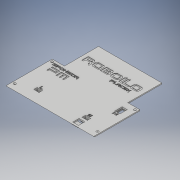
# Autodesk Inventor part: dach
Saved by Autodesk Inventor 2019 (Build 230136000, 136)
## iProperties
Created: 2019-09-08
Part Number: dach
Material: Generic
Document SubType Name: Modeling
Designer: Michal
Density: 1 g/cm^3
Appearance: Default
Author: Michal
Autodesk Inventor part; units mm, degrees
ref_plane "YZ Plane" through (0, 0, 0) normal (1, 0, 0) x (0, 1, 0)
ref_plane "XZ Plane" through (0, 0, 0) normal (0, 1, 0) x (-1, 0, 0)
ref_plane "XY Plane" through (0, 0, 0) normal (0, 0, 1) x (1, 0, 0)
sketch "Sketch1" plane through (0, 0, 0) normal (0, 1, 0) x (-1, 0, 0)
  line L0 (0, 0) -> (180, 0)
  line L1 (180, 0) -> (180, -95)
  line L2 (0, 0) -> (0, -95)
  line L3 (180, -95) -> (155, -95)
  line L4 (0, -95) -> (25, -95)
  line L5 (25, -95) -> (25, -165)
  line L6 (155, -95) -> (155, -165)
  line L7 (155, -165) -> (25, -165)
  dimension "d0" = 180
  dimension "d1" = 95
  dimension "d4" = 95
  dimension "d35" = 25
  dimension "d36" = 25
  constraints: 16 end point, 4 horizontal, 2 perpendicular, 2 vertical
  measures "d0" distance of L0.start L0.end
  measures "d1" distance of L0.end L1.end
  measures "d4" distance of L0.start L2.end
  measures "d35" distance of L1.end L3.end
  measures "d36" distance of L2.end L4.end
extrude "Extrusion1" add sketch "Sketch1" along normal blind 2
sketch "Sketch3" plane through (-155, 0, -165) normal (-1, 0, 0) x (0, 0, 1)
  line L0 (70, 2) -> (0, 2) projected
  line L1 (0, 2) -> (28, 2)
  line L2 (28, 2) -> (28, -13)
  circle A0 centre (28, -13) radius 12.5
  point P0 (165, 0)
  dimension "d46" = 28
  dimension "d47" = 15
  dimension "d48" = 25
  constraints: 4 end point, 1 centre point, 1 coincident, 1 perpendicular, 1 point on line
  measures "d46" distance of L0.end L1.end
  measures "d47" distance of L1.end L2.end
  measures "d48" diameter of A0
extrude "Extrusion3" cut sketch "Sketch3" against normal blind 130
chamfer "Chamfer1" distance 2 angle 45 1 edges at (-90, 0, 0)
sketch "Sketch7" plane through (0, 2, 0) normal (0, 1, 0) x (1, 0, 0)
  line L0 (-155, 95) -> (-180, 95) projected
  line L1 (-180, 95) -> (-175, 95)
  line L2 (-175, 95) -> (-175, 90)
  line L3 (-175, 90) -> (-180, 90)
  line L4 (-180, 90) -> (-180, 95)
  line L5 (0, 95) -> (-25, 95) projected
  line L6 (0, 95) -> (-5, 95)
  line L7 (-5, 95) -> (-5, 90)
  line L8 (-5, 90) -> (0, 90)
  line L9 (0, 90) -> (0, 95)
  line L10 (-5, 90) -> (-5, 13)
  line L11 (-175, 90) -> (-175, 13)
  point P0 (0, 0)
  dimension "d80" = 5
  dimension "d81" = 5
  dimension "d82" = 5
  dimension "d83" = 77
  constraints: 20 end point, 4 parallel, 2 horizontal, 2 perpendicular, 2 vertical, 1 point on line
  measures "d80" distance of L2.end L3.end
  measures "d81" distance of L1.end L2.end
  measures "d82" distance of L8.end L7.end
  measures "d83" distance of L7.end L10.end
hole "Hole1" at (-175, 2, -90) at (-5, 2, -90) at (-5, 2, -13) at (-175, 2, -13) direction (0, -1, 0) diameter 2.4638 depth 8.7884 countersink diameter 5 countersink angle 75
sketch "Sketch8" plane through (0, 2, 0) normal (0, 1, 0) x (1, 0, 0)
  line L0 (0, 0) -> (0, 95) projected
  line L1 (0, 95) -> (-13, 95)
  line L2 (-13, 95) -> (-13, 82)
  line L3 (-13, 82) -> (0, 82)
  line L4 (0, 82) -> (0, 95)
  line L5 (-13, 82) -> (-23.5, 82)
  line L6 (-23.5, 82) -> (-23.5, 67)
  line L7 (-23.5, 67) -> (-13, 67)
  line L8 (-13, 67) -> (-13, 82)
  line L9 (-180, 95) -> (-180, 0) projected
  line L10 (-180, 0) -> (0, 0) projected
  line L11 (0, 0) -> (-35, 0)
  line L12 (-35, 0) -> (-35, 4)
  line L13 (-35, 4) -> (0, 4)
  line L14 (0, 4) -> (0, 0)
  line L15 (-35, 4) -> (-47, 4)
  line L16 (-47, 4) -> (-47, 17)
  line L17 (-47, 17) -> (-35, 17)
  line L18 (-35, 17) -> (-35, 4)
  line L19 (-35, 17) -> (-35, 22)
  line L20 (-35, 22) -> (-46, 22)
  line L21 (-46, 22) -> (-46, 29)
  line L22 (-46, 29) -> (-35, 29)
  line L23 (-35, 29) -> (-35, 22)
  line L24 (-180, 0) -> (-145, 0)
  line L25 (-145, 0) -> (-145, 22)
  line L26 (-145, 22) -> (-180, 22)
  line L27 (-180, 22) -> (-180, 0)
  line L28 (-145, 22) -> (-134, 22)
  line L29 (-134, 22) -> (-134, 29)
  line L30 (-134, 29) -> (-145, 29)
  line L31 (-145, 29) -> (-145, 22)
  dimension "d91" = 13
  dimension "d92" = 13
  dimension "d93" = 10.5
  dimension "d94" = 15
  dimension "d128" = 35
  dimension "d129" = 4
  dimension "d130" = 12
  dimension "d131" = 13
  dimension "d141" = 5
  dimension "d142" = 11
  dimension "d143" = 7
  dimension "d158" = 35
  dimension "d159" = 22
  dimension "d160" = 11
  dimension "d161" = 7
  constraints: 58 end point, 14 parallel, 7 horizontal, 7 perpendicular, 1 vertical
  measures "d91" distance of L3.end L2.end
  measures "d92" distance of L2.end L1.end
  measures "d93" distance of L7.end L6.end
  measures "d94" distance of L6.end L5.end
  measures "d128" distance of L12.end L13.end
  measures "d129" distance of L11.end L12.end
  measures "d130" distance of L16.end L17.end
  measures "d131" distance of L15.end L16.end
  measures "d141" distance of L17.end L19.end
  measures "d142" distance of L21.end L22.end
  measures "d143" distance of L20.end L21.end
  measures "d158" distance of L26.end L25.end
  measures "d159" distance of L25.end L24.end
  measures "d160" distance of L30.end L29.end
  measures "d161" distance of L29.end L28.end
extrude "Extrusion7" cut sketch "Sketch8" against normal blind 2 contours L15 L16 L17 L18 | L8 L7 L6 L5 | L31 L30 L29 L28 | L20 L21 L22 L23
sketch "Sketch9" plane through (0, 0, 0) normal (0, -1, 0) x (1, 0, 0)
  line L0 (-13, -67) -> (-23.5, -67) projected
  line L1 (-23.5, -67) -> (-23.5, -82) projected
  line L2 (-13, -67) -> (-23.5, -67)
  line L3 (-23.5, -67) -> (-23.5, -82)
  line L4 (-23.5, -82) -> (-13, -82)
  line L5 (-13, -82) -> (-13, -67)
  line L6 (-23.5, -82) -> (-13, -82) projected
  line L7 (-11, -65) -> (-25.5, -65)
  line L8 (-25.5, -65) -> (-25.5, -84)
  line L9 (-25.5, -84) -> (-11, -84)
  line L10 (-11, -84) -> (-11, -65)
  point P0 (0, 0)
  constraints: 16 end point, 4 parallel, 2 horizontal, 2 perpendicular
extrude "Extrusion8" add sketch "Sketch9" along normal blind 3
sketch "Sketch10" plane through (-13, 2, -82) normal (-1, 0, 0) x (0, 0, 1)
  line L0 (0, 0) -> (15, 0) projected
  line L1 (0, 0) -> (0, -3)
  line L2 (0, 0) -> (0, -5) projected
  line L3 (15, 0) -> (15, -5) projected
  line L4 (0, -3) -> (15, -3)
  line L5 (15, -3) -> (15, -5)
  line L6 (15, -5) -> (0, -5)
  line L7 (0, -5) -> (0, -3)
  point P0 (82, -2)
  dimension "d103" = 3
  constraints: 10 end point, 2 parallel, 1 horizontal, 1 perpendicular, 1 point on line
  measures "d103" distance of L0.start L1.end
extrude "Extrusion9" add sketch "Sketch10" along normal blind 1 contours L4 L3 L6 L2
sketch "Sketch11" plane through (-23.5, 2, -67) normal (1, 0, 0) x (0, 0, -1)
  line L0 (15, 0) -> (15, -3) projected
  line L1 (15, 0) -> (15, -3)
  line L2 (0, -3) -> (15, -3) projected
  line L3 (15, -5) -> (0, -5) projected
  line L4 (15, -3) -> (0, -3)
  line L5 (0, -3) -> (0, -5)
  line L6 (0, -5) -> (15, -5)
  line L7 (15, -5) -> (15, -3)
  point P0 (-67, -2)
  constraints: 10 end point, 2 parallel, 1 horizontal, 1 perpendicular, 1 vertical
extrude "Extrusion10" add sketch "Sketch11" along normal blind 1
sketch "Sketch12" plane through (-23.5, 2, -82) normal (0, 0, 1) x (1, 0, 0)
  line L0 (9.5, -3) -> (9.5, -5) projected
  line L1 (1, -3) -> (0, -3) projected
  line L2 (9.5, -5) -> (1, -5)
  line L3 (1, -5) -> (1, -3)
  line L4 (1, -3) -> (9.5, -3)
  line L5 (9.5, -3) -> (9.5, -5)
  point P0 (23.5, -2)
  constraints: 8 end point, 2 parallel, 1 horizontal, 1 perpendicular
extrude "Extrusion11" add sketch "Sketch12" along normal blind 1.3
sketch "Sketch13" plane through (-13, 2, -67) normal (0, 0, -1) x (-1, 0, 0)
  line L0 (0, -3) -> (1, -3) projected
  line L1 (-2, -5) -> (12.5, -5) projected
  line L2 (0, -3) -> (10.5024, -3)
  line L3 (10.5024, -3) -> (10.5024, -5)
  line L4 (10.5024, -5) -> (0, -5)
  line L5 (0, -5) -> (0, -3)
  point P0 (-13, -2)
  constraints: 8 end point, 2 parallel, 1 horizontal, 1 perpendicular, 1 point on line
extrude "Extrusion12" add sketch "Sketch13" along normal blind 1.3
sketch "Sketch14" plane through (0, -3, 0) normal (0, -1, 0) x (1, 0, 0)
  line L0 (-22.5, -68.3) -> (-22.5, -67)
  line L1 (-13, -67) -> (-23.5, -67) projected
  line L2 (-22.5, -67) -> (-14, -67)
  line L3 (-22.5, -68.3) -> (-14, -68.3) projected
  line L4 (-14, -67) -> (-14, -68.3)
  line L5 (-14, -68.3) -> (-22.5, -68.3)
  line L6 (-22.5, -80.7) -> (-22.5, -68.3) projected
  line L7 (-22.5, -80.7) -> (-22.5, -82)
  line L8 (-23.5, -82) -> (-13, -82) projected
  line L9 (-14, -80.7) -> (-22.5, -80.7) projected
  line L10 (-22.5, -80.7) -> (-14, -80.7)
  line L11 (-14, -80.7) -> (-14, -82)
  line L12 (-14, -82) -> (-22.5, -82)
  point P0 (0, 0)
  constraints: 16 end point, 3 perpendicular, 2 collinear, 2 point on line, 2 vertical, 1 horizontal
extrude "Extrusion13" cut sketch "Sketch14" against normal blind 1
sketch "Sketch17" plane through (0, 0, 0) normal (0, -1, 0) x (1, 0, 0)
  line L0 (-47, -4) -> (-35, -4) projected
  line L1 (-35, -17) -> (-47, -17) projected
  line L2 (-35, -4) -> (-47, -4)
  line L3 (-47, -4) -> (-47, -17)
  line L4 (-47, -17) -> (-35, -17)
  line L5 (-35, -17) -> (-35, -4)
  line L6 (-34, -4) -> (-34, -3)
  line L7 (-34, -3) -> (-35, -3)
  line L8 (-48, -17) -> (-48, -18)
  line L9 (-48, -18) -> (-47, -18)
  line L10 (-48, -18) -> (-34, -18)
  line L11 (-34, -18) -> (-34, -3)
  line L12 (-34, -3) -> (-48, -3)
  line L13 (-48, -3) -> (-48, -18)
  point P0 (0, 0)
  dimension "d132" = 1
  dimension "d133" = 1
  dimension "d134" = 1
  dimension "d135" = 1
  constraints: 24 end point, 4 parallel, 2 horizontal, 2 perpendicular
  measures "d132" distance of L7.end L6.end
  measures "d133" distance of L6.end L6.start
  measures "d134" distance of L9.end L8.end
  measures "d135" distance of L8.end L8.start
extrude "Extrusion16" add sketch "Sketch17" along normal blind 0.5
sketch "Sketch18" plane through (0, -0.5, 0) normal (0, -1, 0) x (1, 0, 0)
  line L0 (-34, -3) -> (-48, -3) projected
  line L1 (-34, -18) -> (-34, -3) projected
  line L2 (-48, -3) -> (-34, -3)
  line L3 (-34, -3) -> (-34, -13)
  line L4 (-34, -13) -> (-48, -13)
  line L5 (-48, -13) -> (-48, -3)
  point P0 (0, 0)
  dimension "d138" = 10
  constraints: 8 end point, 2 parallel, 1 horizontal, 1 perpendicular, 1 point on line
  measures "d138" distance of L2.end L3.end
extrude "Extrusion17" add sketch "Sketch18" along normal blind 1
sketch "Sketch19" plane through (0, 0, 0) normal (0, -1, 0) x (1, 0, 0)
  line L0 (-46, -22) -> (-35, -22) projected
  line L1 (-35, -22) -> (-46, -22)
  line L2 (-46, -22) -> (-46, -29)
  line L3 (-46, -29) -> (-35, -29)
  line L4 (-35, -29) -> (-35, -22)
  line L5 (-47, -30) -> (-34, -30)
  line L6 (-34, -30) -> (-34, -21)
  line L7 (-34, -21) -> (-47, -21)
  line L8 (-47, -21) -> (-47, -30)
  line L9 (-134, -22) -> (-145, -22)
  line L10 (-145, -22) -> (-145, -29)
  line L11 (-145, -29) -> (-134, -29)
  line L12 (-134, -29) -> (-134, -22)
  line L13 (-146, -30) -> (-133, -30)
  line L14 (-133, -30) -> (-133, -21)
  line L15 (-133, -21) -> (-146, -21)
  line L16 (-146, -21) -> (-146, -30)
  point P0 (0, 0)
  constraints: 32 end point, 8 parallel, 4 horizontal, 4 perpendicular
extrude "Extrusion18" add sketch "Sketch19" along normal blind 4
sketch "Sketch20" plane through (0, -4, 0) normal (0, -1, 0) x (1, 0, 0)
  line L0 (-34, -30) -> (-47, -30) projected
  line L1 (-47, -21) -> (-34, -21) projected
  line L2 (-34, -30) -> (-47, -30)
  line L3 (-47, -30) -> (-47, -21)
  line L4 (-47, -21) -> (-34, -21)
  line L5 (-34, -21) -> (-34, -30)
  line L6 (-46, -22) -> (-46, -29) projected
  line L7 (-46, -29) -> (-35, -29) projected
  line L8 (-46, -22) -> (-42, -22)
  line L9 (-42, -22) -> (-42, -29)
  line L10 (-42, -29) -> (-46, -29)
  line L11 (-46, -29) -> (-46, -22)
  line L12 (-35, -22) -> (-46, -22) projected
  line L13 (-35, -29) -> (-39, -29)
  line L14 (-39, -29) -> (-39, -22)
  line L15 (-39, -22) -> (-35, -22)
  line L16 (-35, -22) -> (-35, -29)
  line L17 (-133, -30) -> (-146, -30) projected
  line L18 (-133, -30) -> (-146, -30)
  line L19 (-146, -30) -> (-146, -21)
  line L20 (-146, -21) -> (-133, -21)
  line L21 (-133, -21) -> (-133, -30)
  line L22 (-145, -22) -> (-141, -22)
  line L23 (-141, -22) -> (-141, -29)
  line L24 (-141, -29) -> (-145, -29)
  line L25 (-145, -29) -> (-145, -22)
  line L26 (-134, -29) -> (-138, -29)
  line L27 (-138, -29) -> (-138, -22)
  line L28 (-138, -22) -> (-134, -22)
  line L29 (-134, -22) -> (-134, -29)
  point P0 (0, 0)
  dimension "d150" = 4
  dimension "d151" = 4
  dimension "d162" = 4
  dimension "d163" = 4
  constraints: 48 end point, 12 parallel, 6 horizontal, 6 perpendicular, 2 point on line
  measures "d150" distance of L9.end L10.end
  measures "d151" distance of L14.end L15.end
  measures "d162" distance of L23.end L25.start
  measures "d163" distance of L28.start L29.start
extrude "Extrusion19" add sketch "Sketch20" along normal blind 1.5 contours L0 L3 L1 L5 | L12 L14 L7 L9 | L17 L19 L20 L21
sketch "Sketch5" plane through (0, 2, 0) normal (0, 1, 0) x (1, 0, 0)
  line L0 (-154.7367, 165.2131) -> (-24.9468, 165.2131) construction
  line L1 (-24.9468, 165.2131) -> (-24.9468, 95.1481) construction
  line L2 (-24.9468, 95.1481) -> (-154.7367, 95.1481) construction
  line L3 (-154.7367, 95.1481) -> (-154.7367, 165.2131) construction
  line L4 (-82.3644, 120.7847) -> (-41.6119, 120.7847) construction
  line L5 (-41.6119, 120.7847) -> (-41.6119, 113.7771) construction
  line L6 (-41.6119, 113.7771) -> (-82.3644, 113.7771) construction
  line L7 (-82.3644, 113.7771) -> (-82.3644, 120.7847) construction
  line L8 (-44.6378, 36.0437) -> (-36.7668, 36.0437) construction
  line L9 (-36.7668, 36.0437) -> (-36.7668, 30.8473) construction
  line L10 (-36.7668, 30.8473) -> (-44.6378, 30.8473) construction
  line L11 (-44.6378, 30.8473) -> (-44.6378, 36.0437) construction
  line L12 (-22.1506, 65.5798) -> (-13.2194, 65.5798) construction
  line L13 (-13.2194, 65.5798) -> (-13.2194, 59.4838) construction
  line L14 (-13.2194, 59.4838) -> (-22.1506, 59.4838) construction
  line L15 (-22.1506, 59.4838) -> (-22.1506, 65.5798) construction
  line L16 (-142.4189, 36.7707) -> (-136.2064, 36.7707) construction
  line L17 (-136.2064, 36.7707) -> (-136.2064, 30.6546) construction
  line L18 (-136.2064, 30.6546) -> (-142.4189, 30.6546) construction
  line L19 (-142.4189, 30.6546) -> (-142.4189, 36.7707) construction
  line L20 (-180, 2) -> (-180, 95) projected
  line L21 (-166.0933, 81.4189) -> (-150.8913, 81.4189)
  line L22 (-150.8913, 81.4189) -> (-150.8913, 72.9559)
  line L23 (-166.0933, 81.4189) -> (-166.0933, 78.7799)
  line L24 (-166.0933, 78.7799) -> (-153.5243, 78.7799)
  line L25 (-153.5243, 78.7799) -> (-153.5243, 75.5879)
  line L26 (-153.5243, 75.5879) -> (-166.0933, 75.5879)
  line L27 (-166.0933, 75.5879) -> (-166.0933, 69.8939)
  line L28 (-166.0933, 69.8939) -> (-163.4573, 69.8939)
  line L29 (-163.4573, 69.8939) -> (-163.4573, 72.9559)
  line L30 (-163.4573, 72.9559) -> (-150.8913, 72.9559)
  line L31 (-150.8913, 81.4189) -> (-147.5843, 81.4189)
  line L32 (-147.5843, 81.4189) -> (-147.5843, 69.8939)
  line L33 (-147.5843, 69.8939) -> (-144.9503, 69.8939)
  line L34 (-144.9503, 69.8939) -> (-144.9503, 78.7799)
  line L35 (-144.9503, 78.7799) -> (-133.8883, 78.7799)
  line L36 (-133.8883, 78.7799) -> (-133.8883, 69.8939)
  line L37 (-133.8883, 69.8939) -> (-131.2543, 69.8939)
  line L38 (-131.2543, 69.8939) -> (-131.2543, 81.4189)
  line L39 (-131.2543, 81.4189) -> (-147.5843, 81.4189)
  line L40 (-144.9503, 78.7799) -> (-140.7343, 78.7799)
  line L41 (-133.8883, 78.7799) -> (-138.1043, 78.7799)
  line L42 (-138.1043, 78.7799) -> (-138.1043, 77.2269)
  line L43 (-138.1043, 77.2269) -> (-140.7343, 77.2269)
  line L44 (-140.7343, 77.2269) -> (-140.7343, 69.8939)
  line L45 (-140.7343, 69.8939) -> (-138.1043, 69.8939)
  line L46 (-138.1043, 69.8939) -> (-138.1043, 77.2269)
  line L47 (-170.8643, 90.9845) -> (-118.0724, 90.9845) construction
  line L48 (-118.0724, 90.9845) -> (-118.0724, 83.2717) construction
  line L49 (-118.0724, 83.2717) -> (-170.8643, 83.2717) construction
  line L50 (-170.8643, 83.2717) -> (-170.8643, 90.9845) construction
  line L51 (-75.7423, 118.2788) -> (-77.1197, 116.4155)
  line L52 (-77.1197, 116.4155) -> (-80.7902, 116.4155)
  line L53 (-80.7902, 116.4155) -> (-80.7902, 113.7771)
  line L54 (-80.7902, 113.7771) -> (-82.3604, 114.6766)
  line L55 (-82.3604, 114.6766) -> (-82.3604, 119.8731)
  line L56 (-82.3604, 119.8731) -> (-76.927, 119.8731)
  line L57 (-76.927, 119.8731) -> (-75.7423, 118.2788)
  line L58 (-77.3607, 118.1704) -> (-77.7743, 118.7165)
  line L59 (-77.7743, 118.7165) -> (-80.7902, 118.7165)
  line L60 (-80.7902, 118.7165) -> (-80.7902, 117.5961)
  line L61 (-80.7902, 117.5961) -> (-77.7743, 117.5961)
  line L62 (-77.7743, 117.5961) -> (-77.3607, 118.1704)
  line L63 (-69.1925, 115.8332) -> (-70.3571, 114.6686)
  line L64 (-70.3571, 114.6686) -> (-75.2283, 114.6686)
  line L65 (-75.2283, 114.6686) -> (-75.2283, 119.8771)
  line L66 (-75.2283, 119.8771) -> (-73.6581, 120.7847)
  line L67 (-73.6581, 120.7847) -> (-73.6581, 115.8332)
  line L68 (-73.6581, 115.8332) -> (-69.1925, 115.8332)
  line L69 (-62.707, 113.7771) -> (-64.2852, 114.6686)
  line L70 (-64.2852, 114.6686) -> (-64.2852, 116.1665)
  line L71 (-64.2852, 116.1665) -> (-67.4456, 116.1665)
  line L72 (-67.4456, 116.1665) -> (-67.4456, 114.6686)
  line L73 (-67.4456, 114.6686) -> (-69.0158, 114.6766)
  line L74 (-69.0158, 114.6766) -> (-69.0158, 118.7085)
  line L75 (-69.0158, 118.7085) -> (-67.8352, 119.8731)
  line L76 (-67.8352, 119.8731) -> (-63.8876, 119.8731)
  line L77 (-63.8876, 119.8731) -> (-62.707, 118.7085)
  line L78 (-62.707, 118.7085) -> (-62.707, 113.7771)
  line L79 (-64.2852, 117.315) -> (-64.2852, 118.7085)
  line L80 (-64.2852, 118.7085) -> (-67.4456, 118.7085)
  line L81 (-67.4456, 118.7085) -> (-67.4456, 117.315)
  line L82 (-67.4456, 117.315) -> (-64.2852, 117.315)
  line L83 (-55.5789, 119.8731) -> (-56.7355, 118.7085)
  line L84 (-56.7355, 118.7085) -> (-60.2292, 118.7085)
  line L85 (-60.2292, 118.7085) -> (-60.2292, 115.8332)
  line L86 (-60.2292, 115.8332) -> (-55.7636, 115.8332)
  line L87 (-55.7636, 115.8332) -> (-56.9282, 114.6686)
  line L88 (-56.9282, 114.6686) -> (-60.6188, 114.6686)
  line L89 (-60.6188, 114.6686) -> (-61.7994, 115.8332)
  line L90 (-61.7994, 115.8332) -> (-61.7994, 118.6844)
  line L91 (-61.7994, 118.6844) -> (-60.6188, 119.8731)
  line L92 (-60.6188, 119.8731) -> (-55.5789, 119.8731)
  line L93 (-49.005, 119.8731) -> (-50.1616, 118.7085)
  line L94 (-50.1616, 118.7085) -> (-53.6553, 118.7085)
  line L95 (-53.6553, 118.7085) -> (-53.6553, 117.8009)
  line L96 (-53.6553, 117.8009) -> (-49.764, 117.8009)
  line L97 (-49.764, 117.8009) -> (-50.8242, 116.7407)
  line L98 (-50.8242, 116.7407) -> (-53.6553, 116.7407)
  line L99 (-53.6553, 116.7407) -> (-53.6553, 115.8332)
  line L100 (-53.6553, 115.8332) -> (-49.1898, 115.8332)
  line L101 (-49.1898, 115.8332) -> (-50.3544, 114.6686)
  line L102 (-50.3544, 114.6686) -> (-55.2255, 114.6686)
  line L103 (-55.2255, 114.6686) -> (-55.2255, 119.8731)
  line L104 (-55.2255, 119.8731) -> (-49.005, 119.8731)
  line L105 (-42.3549, 119.8731) -> (-44.3347, 117.9816)
  line L106 (-44.3347, 117.9816) -> (-42.5195, 116.1665)
  line L107 (-42.5195, 116.1665) -> (-42.5195, 114.6686)
  line L108 (-42.5195, 114.6686) -> (-44.0897, 113.7771)
  line L109 (-44.0897, 113.7771) -> (-44.0897, 115.9376)
  line L110 (-44.0897, 115.9376) -> (-45.2503, 117.0981)
  line L111 (-45.2503, 117.0981) -> (-46.9208, 115.528)
  line L112 (-46.9208, 115.528) -> (-46.9208, 114.6686)
  line L113 (-46.9208, 114.6686) -> (-48.491, 114.6766)
  line L114 (-48.491, 114.6766) -> (-48.491, 119.8731)
  line L115 (-48.491, 119.8731) -> (-46.9208, 119.8731)
  line L116 (-46.9208, 119.8731) -> (-46.9208, 117.323)
  line L117 (-46.9208, 117.323) -> (-44.2102, 119.8731)
  line L118 (-44.2102, 119.8731) -> (-42.3549, 119.8731)
  line L119 (-131.1694, 121.4211) -> (-135.0949, 123.67)
  line L120 (-135.0949, 123.67) -> (-135.0949, 126.8525)
  line L121 (-135.0949, 126.8525) -> (-136.2896, 128.0171)
  line L122 (-136.2896, 128.0171) -> (-143.7891, 128.0171)
  line L123 (-143.7891, 128.0171) -> (-143.7891, 123.67)
  line L124 (-143.7891, 123.67) -> (-147.7146, 123.67)
  line L125 (-147.7146, 123.67) -> (-147.7146, 136.6611)
  line L126 (-147.7146, 136.6611) -> (-134.1311, 136.6611)
  line L127 (-134.1311, 136.6611) -> (-131.1694, 132.6754)
  line L128 (-131.1694, 132.6754) -> (-133.4183, 129.6535)
  line L129 (-133.4183, 129.6535) -> (-131.1694, 127.3946)
  line L130 (-131.1694, 127.3946) -> (-131.1694, 121.4211)
  line L131 (-135.2053, 132.4044) -> (-136.2494, 133.7697)
  line L132 (-136.2494, 133.7697) -> (-143.7891, 133.7697)
  line L133 (-143.7891, 133.7697) -> (-143.7891, 130.9687)
  line L134 (-143.7891, 130.9687) -> (-136.2595, 130.9687)
  line L135 (-136.2595, 130.9687) -> (-135.2053, 132.4044)
  line L136 (-112.1947, 126.6216) -> (-115.1464, 123.67)
  line L137 (-115.1464, 123.67) -> (-125.989, 123.67)
  line L138 (-125.989, 123.67) -> (-128.9407, 126.6216)
  line L139 (-128.9407, 126.6216) -> (-128.9407, 133.7095)
  line L140 (-128.9407, 133.7095) -> (-125.989, 136.6611)
  line L141 (-125.989, 136.6611) -> (-115.1464, 136.6611)
  line L142 (-115.1464, 136.6611) -> (-112.1947, 133.7095)
  line L143 (-112.1947, 133.7095) -> (-112.1947, 126.6216)
  line L144 (-116.1202, 126.5614) -> (-116.1202, 133.7697)
  line L145 (-116.1202, 133.7697) -> (-125.0152, 133.7697)
  line L146 (-125.0152, 133.7697) -> (-125.0152, 126.5614)
  line L147 (-125.0152, 126.5614) -> (-116.1202, 126.5614)
  line L148 (-93.3807, 127.6456) -> (-96.3323, 123.6499)
  line L149 (-96.3323, 123.6499) -> (-110.0965, 123.6499)
  line L150 (-110.0965, 123.6499) -> (-110.0965, 136.6611)
  line L151 (-110.0965, 136.6611) -> (-96.3323, 136.6611)
  line L152 (-96.3323, 136.6611) -> (-93.3807, 132.6654)
  line L153 (-93.3807, 132.6654) -> (-95.2279, 130.1555)
  line L154 (-95.2279, 130.1555) -> (-93.3807, 127.6456)
  line L155 (-97.6776, 127.6456) -> (-98.6313, 128.8303)
  line L156 (-98.6313, 128.8303) -> (-106.171, 128.8303)
  line L157 (-106.171, 128.8303) -> (-106.171, 126.5614)
  line L158 (-106.171, 126.5614) -> (-98.6313, 126.5614)
  line L159 (-98.6313, 126.5614) -> (-97.6776, 127.6456)
  line L160 (-97.6776, 132.6654) -> (-98.6313, 133.7497)
  line L161 (-98.6313, 133.7497) -> (-106.171, 133.7497)
  line L162 (-106.171, 133.7497) -> (-106.171, 131.4807)
  line L163 (-106.171, 131.4807) -> (-98.6313, 131.4807)
  line L164 (-98.6313, 131.4807) -> (-97.6776, 132.6654)
  line L165 (-74.5766, 126.6216) -> (-77.5283, 123.67)
  line L166 (-77.5283, 123.67) -> (-88.3709, 123.67)
  line L167 (-88.3709, 123.67) -> (-91.3226, 126.6216)
  line L168 (-91.3226, 126.6216) -> (-91.3226, 133.7095)
  line L169 (-91.3226, 133.7095) -> (-88.3709, 136.6611)
  line L170 (-88.3709, 136.6611) -> (-77.5283, 136.6611)
  line L171 (-77.5283, 136.6611) -> (-74.5766, 133.7095)
  line L172 (-74.5766, 133.7095) -> (-74.5766, 126.6216)
  line L173 (-78.5021, 126.5614) -> (-78.5021, 133.7697)
  line L174 (-78.5021, 133.7697) -> (-87.3971, 133.7697)
  line L175 (-87.3971, 133.7697) -> (-87.3971, 126.5614)
  line L176 (-87.3971, 126.5614) -> (-78.5021, 126.5614)
  line L177 (-68.5529, 123.6499) -> (-72.4784, 123.67)
  line L178 (-72.4784, 123.67) -> (-72.4784, 136.6712)
  line L179 (-72.4784, 136.6712) -> (-68.5529, 138.9401)
  line L180 (-68.5529, 138.9401) -> (-68.5529, 123.6499)
  line L181 (-51.2347, 126.5614) -> (-54.1462, 123.6499)
  line L182 (-54.1462, 123.6499) -> (-66.3241, 123.6499)
  line L183 (-66.3241, 123.6499) -> (-66.3241, 136.6712)
  line L184 (-66.3241, 136.6712) -> (-62.3987, 138.9401)
  line L185 (-62.3987, 138.9401) -> (-62.3987, 126.5614)
  line L186 (-62.3987, 126.5614) -> (-51.2347, 126.5614)
  line L187 (-34.0471, 126.6216) -> (-36.9987, 123.67)
  line L188 (-36.9987, 123.67) -> (-47.8414, 123.67)
  line L189 (-47.8414, 123.67) -> (-50.793, 126.6216)
  line L190 (-50.793, 126.6216) -> (-50.793, 133.7095)
  line L191 (-50.793, 133.7095) -> (-47.8414, 136.6611)
  line L192 (-47.8414, 136.6611) -> (-36.9987, 136.6611)
  line L193 (-36.9987, 136.6611) -> (-34.0471, 133.7095)
  line L194 (-34.0471, 133.7095) -> (-34.0471, 126.6216)
  line L195 (-37.9725, 126.5614) -> (-37.9725, 133.7697)
  line L196 (-37.9725, 133.7697) -> (-46.8675, 133.7697)
  line L197 (-46.8675, 133.7697) -> (-46.8675, 126.5614)
  line L198 (-46.8675, 126.5614) -> (-37.9725, 126.5614)
  line L199 (-14.0989, 60.3834) -> (-15.6691, 60.3834)
  line L200 (-15.6691, 60.3834) -> (-15.6691, 63.7085)
  line L201 (-15.6691, 63.7085) -> (-17.6207, 61.0299)
  line L202 (-17.6207, 61.0299) -> (-18.6367, 61.0299)
  line L203 (-18.6367, 61.0299) -> (-20.5764, 63.7085)
  line L204 (-20.5764, 63.7085) -> (-20.5764, 60.3834)
  line L205 (-20.5764, 60.3834) -> (-22.1466, 59.4838)
  line L206 (-22.1466, 59.4838) -> (-22.1466, 65.5798)
  line L207 (-22.1466, 65.5798) -> (-20.3716, 65.5798)
  line L208 (-20.3716, 65.5798) -> (-18.1227, 62.4877)
  line L209 (-18.1227, 62.4877) -> (-15.8819, 65.5798)
  line L210 (-15.8819, 65.5798) -> (-14.0989, 65.5798)
  line L211 (-14.0989, 65.5798) -> (-14.0989, 60.3834)
  line L212 (-37.4174, 32.4455) -> (-38.598, 30.8473)
  line L213 (-38.598, 30.8473) -> (-44.6338, 30.8473)
  line L214 (-44.6338, 30.8473) -> (-43.4772, 32.0038)
  line L215 (-43.4772, 32.0038) -> (-39.5177, 32.0038)
  line L216 (-39.5177, 32.0038) -> (-39.1482, 32.4455)
  line L217 (-39.1482, 32.4455) -> (-39.5136, 32.9114)
  line L218 (-39.5136, 32.9114) -> (-43.4853, 32.9114)
  line L219 (-43.4853, 32.9114) -> (-44.6338, 34.4454)
  line L220 (-44.6338, 34.4454) -> (-43.4531, 36.0437)
  line L221 (-43.4531, 36.0437) -> (-37.4174, 36.0437)
  line L222 (-37.4174, 36.0437) -> (-38.582, 34.8872)
  line L223 (-38.582, 34.8872) -> (-42.5335, 34.8872)
  line L224 (-42.5335, 34.8872) -> (-42.915, 34.4454)
  line L225 (-42.915, 34.4454) -> (-42.5335, 33.9796)
  line L226 (-42.5335, 33.9796) -> (-38.5619, 33.9796)
  line L227 (-38.5619, 33.9796) -> (-37.4174, 32.4455)
  line L228 (-136.3791, 31.8192) -> (-137.5437, 30.6546)
  line L229 (-137.5437, 30.6546) -> (-142.4149, 30.6546)
  line L230 (-142.4149, 30.6546) -> (-142.4149, 35.8631)
  line L231 (-142.4149, 35.8631) -> (-140.8447, 36.7707)
  line L232 (-140.8447, 36.7707) -> (-140.8447, 31.8192)
  line L233 (-140.8447, 31.8192) -> (-136.3791, 31.8192)
  line L234 (-163.6438, 86.4747) -> (-164.8245, 84.8764)
  line L235 (-164.8245, 84.8764) -> (-170.8603, 84.8764)
  line L236 (-170.8603, 84.8764) -> (-169.7037, 86.033)
  line L237 (-169.7037, 86.033) -> (-165.7441, 86.033)
  line L238 (-165.7441, 86.033) -> (-165.3747, 86.4747)
  line L239 (-165.3747, 86.4747) -> (-165.7401, 86.9405)
  line L240 (-165.7401, 86.9405) -> (-169.7117, 86.9405)
  line L241 (-169.7117, 86.9405) -> (-170.8603, 88.4746)
  line L242 (-170.8603, 88.4746) -> (-169.6796, 90.0729)
  line L243 (-169.6796, 90.0729) -> (-163.6438, 90.0729)
  line L244 (-163.6438, 90.0729) -> (-164.8084, 88.9163)
  line L245 (-164.8084, 88.9163) -> (-168.76, 88.9163)
  line L246 (-168.76, 88.9163) -> (-169.1415, 88.4746)
  line L247 (-169.1415, 88.4746) -> (-168.76, 88.0087)
  line L248 (-168.76, 88.0087) -> (-164.7884, 88.0087)
  line L249 (-164.7884, 88.0087) -> (-163.6438, 86.4747)
  line L250 (-156.3712, 88.4786) -> (-157.7486, 86.6153)
  line L251 (-157.7486, 86.6153) -> (-161.4191, 86.6153)
  line L252 (-161.4191, 86.6153) -> (-161.4191, 83.9769)
  line L253 (-161.4191, 83.9769) -> (-162.9893, 84.8764)
  line L254 (-162.9893, 84.8764) -> (-162.9893, 90.0729)
  line L255 (-162.9893, 90.0729) -> (-157.5559, 90.0729)
  line L256 (-157.5559, 90.0729) -> (-156.3712, 88.4786)
  line L257 (-157.9896, 88.3702) -> (-158.4032, 88.9163)
  line L258 (-158.4032, 88.9163) -> (-161.4191, 88.9163)
  line L259 (-161.4191, 88.9163) -> (-161.4191, 87.7959)
  line L260 (-161.4191, 87.7959) -> (-158.4032, 87.7959)
  line L261 (-158.4032, 87.7959) -> (-157.9896, 88.3702)
  line L262 (-149.1588, 86.0571) -> (-150.3395, 84.8764)
  line L263 (-150.3395, 84.8764) -> (-154.6765, 84.8764)
  line L264 (-154.6765, 84.8764) -> (-155.8572, 86.0571)
  line L265 (-155.8572, 86.0571) -> (-155.8572, 88.8922)
  line L266 (-155.8572, 88.8922) -> (-154.6765, 90.0729)
  line L267 (-154.6765, 90.0729) -> (-150.3395, 90.0729)
  line L268 (-150.3395, 90.0729) -> (-149.1588, 88.8922)
  line L269 (-149.1588, 88.8922) -> (-149.1588, 86.0571)
  line L270 (-150.729, 86.033) -> (-150.729, 88.9163)
  line L271 (-150.729, 88.9163) -> (-154.287, 88.9163)
  line L272 (-154.287, 88.9163) -> (-154.287, 86.033)
  line L273 (-154.287, 86.033) -> (-150.729, 86.033)
  line L274 (-141.8701, 84.8764) -> (-143.0628, 84.8764)
  line L275 (-143.0628, 84.8764) -> (-146.7493, 87.9124)
  line L276 (-146.7493, 87.9124) -> (-146.7493, 84.8764)
  line L277 (-146.7493, 84.8764) -> (-148.3195, 84.8844)
  line L278 (-148.3195, 84.8844) -> (-148.3195, 90.0729)
  line L279 (-148.3195, 90.0729) -> (-147.1991, 90.0729)
  line L280 (-147.1991, 90.0729) -> (-143.4403, 86.9767)
  line L281 (-143.4403, 86.9767) -> (-143.4403, 90.0769)
  line L282 (-143.4403, 90.0769) -> (-141.8701, 90.9845)
  line L283 (-141.8701, 90.9845) -> (-141.8701, 84.8764)
  line L284 (-133.7702, 86.4747) -> (-134.9509, 84.8764)
  line L285 (-134.9509, 84.8764) -> (-140.9866, 84.8764)
  line L286 (-140.9866, 84.8764) -> (-139.8301, 86.033)
  line L287 (-139.8301, 86.033) -> (-135.8705, 86.033)
  line L288 (-135.8705, 86.033) -> (-135.501, 86.4747)
  line L289 (-135.501, 86.4747) -> (-135.8665, 86.9405)
  line L290 (-135.8665, 86.9405) -> (-139.8381, 86.9405)
  line L291 (-139.8381, 86.9405) -> (-140.9866, 88.4746)
  line L292 (-140.9866, 88.4746) -> (-139.806, 90.0729)
  line L293 (-139.806, 90.0729) -> (-133.7702, 90.0729)
  line L294 (-133.7702, 90.0729) -> (-134.9348, 88.9163)
  line L295 (-134.9348, 88.9163) -> (-138.8864, 88.9163)
  line L296 (-138.8864, 88.9163) -> (-139.2679, 88.4746)
  line L297 (-139.2679, 88.4746) -> (-138.8864, 88.0087)
  line L298 (-138.8864, 88.0087) -> (-134.9147, 88.0087)
  line L299 (-134.9147, 88.0087) -> (-133.7702, 86.4747)
  line L300 (-126.4173, 86.0571) -> (-127.5979, 84.8764)
  line L301 (-127.5979, 84.8764) -> (-131.935, 84.8764)
  line L302 (-131.935, 84.8764) -> (-133.1157, 86.0571)
  line L303 (-133.1157, 86.0571) -> (-133.1157, 88.8922)
  line L304 (-133.1157, 88.8922) -> (-131.935, 90.0729)
  line L305 (-131.935, 90.0729) -> (-127.5979, 90.0729)
  line L306 (-127.5979, 90.0729) -> (-126.4173, 88.8922)
  line L307 (-126.4173, 88.8922) -> (-126.4173, 86.0571)
  line L308 (-127.9875, 86.033) -> (-127.9875, 88.9163)
  line L309 (-127.9875, 88.9163) -> (-131.5455, 88.9163)
  line L310 (-131.5455, 88.9163) -> (-131.5455, 86.033)
  line L311 (-131.5455, 86.033) -> (-127.9875, 86.033)
  line L312 (-118.9599, 83.9769) -> (-120.5301, 84.8764)
  line L313 (-120.5301, 84.8764) -> (-120.5301, 86.1494)
  line L314 (-120.5301, 86.1494) -> (-121.008, 86.6153)
  line L315 (-121.008, 86.6153) -> (-124.0078, 86.6153)
  line L316 (-124.0078, 86.6153) -> (-124.0078, 84.8764)
  line L317 (-124.0078, 84.8764) -> (-125.578, 84.8764)
  line L318 (-125.578, 84.8764) -> (-125.578, 90.0729)
  line L319 (-125.578, 90.0729) -> (-120.1446, 90.0729)
  line L320 (-120.1446, 90.0729) -> (-118.9599, 88.4786)
  line L321 (-118.9599, 88.4786) -> (-119.8595, 87.2698)
  line L322 (-119.8595, 87.2698) -> (-118.9599, 86.3663)
  line L323 (-118.9599, 86.3663) -> (-118.9599, 83.9769)
  line L324 (-120.5743, 88.3702) -> (-120.9919, 88.9163)
  line L325 (-120.9919, 88.9163) -> (-124.0078, 88.9163)
  line L326 (-124.0078, 88.9163) -> (-124.0078, 87.7959)
  line L327 (-124.0078, 87.7959) -> (-120.9959, 87.7959)
  line L328 (-120.9959, 87.7959) -> (-120.5743, 88.3702)
  point P0 (0, 0)
  dimension "d166" = 15.202
  dimension "d167" = 8.463
  dimension "d168" = 2.639
  dimension "d169" = 12.569
  dimension "d170" = 3.192
  dimension "d171" = 5.694
  dimension "d172" = 2.636
  dimension "d173" = 3.307
  dimension "d174" = 2.634
  dimension "d175" = 8.886
  dimension "d176" = 11.062
  dimension "d177" = 2.634
  dimension "d178" = 4.216
  dimension "d179" = 4.216
  dimension "d180" = 1.553
  constraints: 52 end point, 15 perpendicular, 7 point on line, 3 horizontal, 3 parallel, 1 vertical, 12 other
  measures "d166" distance of L21.start L21.end
  measures "d167" distance of L21.end L22.end
  measures "d168" distance of L21.start L23.end
  measures "d169" distance of L23.end L24.end
  measures "d170" distance of L24.end L25.end
  measures "d171" distance of L26.end L27.end
  measures "d172" distance of L27.end L28.end
  measures "d173" distance of L21.end L31.end
  measures "d174" distance of L32.end L33.end
  measures "d175" distance of L33.end L34.end
  measures "d176" distance of L34.end L35.end
  measures "d177" distance of L36.end L37.end
  measures "d178" distance of L34.end L40.end
  measures "d179" distance of L35.end L41.end
  measures "d180" distance of L41.end L42.end
extrude "Extrusion6" cut sketch "Sketch5" against normal blind 1
body "Solid1"
